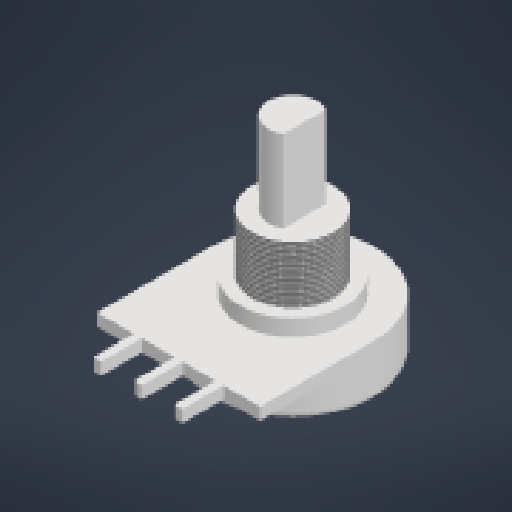
# Autodesk Inventor part: PotMeter
Saved by Autodesk Inventor 2026.1 (Build 301233000, 233)
## iProperties
Created: 2025-11-11
Part Number: PotMeter
Material: Generic
Document SubType Name: Modeling
Designer: Mikke
Density: 1 g/cm^3
Appearance: Default
Author: Mikke
Autodesk Inventor part; units mm, degrees
ref_plane "YZ Plane" through (0, 0, 0) normal (1, 0, 0) x (0, 1, 0)
ref_plane "XZ Plane" through (0, 0, 0) normal (0, 1, 0) x (-1, 0, 0)
ref_plane "XY Plane" through (0, 0, 0) normal (0, 0, 1) x (1, 0, 0)
sketch "Sketch1" plane through (0, 0, 0) normal (0, 1, 0) x (-1, 0, 0)
  circle A0 centre (0, 0) radius 10
  line L0 (10, 0) -> (-10, 0)
  line L1 (-10, 0) -> (-10, 14)
  line L2 (-10, 14) -> (10, 14)
  line L3 (10, 14) -> (10, 0)
  line L4 (-5.5, 14) -> (-4.5, 14)
  line L5 (-0.5, 14) -> (0.5, 14)
  line L6 (4.5, 14) -> (5.5, 14)
  line L7 (5.5, 14) -> (4.5, 14)
  line L8 (4.5, 14) -> (4.5, 19)
  line L9 (4.5, 19) -> (5.5, 19)
  line L10 (5.5, 19) -> (5.5, 14)
  line L11 (0.5, 14) -> (-0.5, 14)
  line L12 (-0.5, 14) -> (-0.5, 19)
  line L13 (-0.5, 19) -> (0.5, 19)
  line L14 (0.5, 19) -> (0.5, 14)
  line L15 (-4.5, 14) -> (-5.5, 14)
  line L16 (-5.5, 14) -> (-5.5, 19)
  line L17 (-5.5, 19) -> (-4.5, 19)
  line L18 (-4.5, 19) -> (-4.5, 14)
  point P0 (0, 14)
  point P1 (5, 14)
  point P2 (-5, 14)
  dimension "d0" = 20
  dimension "d1" = 20
  dimension "d2" = 14
  dimension "d5" = 1
  dimension "d6" = 1
  dimension "d7" = 1
  dimension "d8" = 5
  dimension "d9" = 5
  dimension "d10" = 5
  constraints: 38 end point, 8 parallel, 7 coincident, 5 point on line, 4 horizontal, 4 midpoint, 4 perpendicular, 3 other
  measures "d1" distance of L1.end L2.end
  measures "d2" distance of L0.end L1.end
  measures "d5" distance of L4.start L4.end
  measures "d6" distance of L5.start L5.end
  measures "d7" distance of L6.start L6.end
  measures "d8" distance of L7.end L8.end
  measures "d9" distance of L11.end L12.end
  measures "d10" distance of L15.end L16.end
extrude "Extrusion1" add sketch "Sketch1" along normal blind 1.5
sketch "Sketch2" plane through (0, 0, 0) normal (0, -1, 0) x (1, 0, 0)
  circle A0 centre (0, 0) radius 10
  constraints: 1 centre point, 1 coincident
extrude "Extrusion2" add sketch "Sketch2" along normal blind 5
sketch "Sketch3" plane through (0, 1.5, 0) normal (0, 1, 0) x (1, 0, 0)
  circle A0 centre (0, 0) radius 6.5
  dimension "d13" = 13
  constraints: 1 centre point, 1 coincident
  measures "d13" diameter of A0
extrude "Extrusion3" add sketch "Sketch3" along normal blind 2
sketch "Sketch4" plane through (0, 3.5, 0) normal (0, 1, 0) x (1, 0, 0)
  circle A0 centre (0, 0) radius 5
  dimension "d16" = 10
  constraints: 1 centre point, 1 coincident
  measures "d16" diameter of A0
extrude "Extrusion4" add sketch "Sketch4" along normal blind 7
thread "Thread1" size "M3x0.5" class "6g" standard "ANSI Metric M Profile" full length
sketch "Sketch5" plane through (0, 10.5, 0) normal (0, 1, 0) x (1, 0, 0)
  circle A0 centre (0, 0) radius 3
  line L0 (0, 0) -> (1.5, 0)
  line L1 (1.5, -2.5981) -> (1.5, 2.5981)
  point P0 (0.0162, 1.5)
  point P1 (-2.4, 1.8)
  dimension "d21" = 6
  dimension "d27" = 1.5
  constraints: 4 end point, 2 point on circle, 1 centre point, 1 coincident, 1 horizontal, 1 midpoint, 1 vertical
  measures "d21" diameter of A0
  measures "d27" distance of L0.start L0.end
extrude "Extrusion5" add sketch "Sketch5" along normal blind 10 contours L1 A0 picked at (-1.4848, 0)
fillet "Fillet1" radius 1 1 edges at (-10, -5, 0)
fillet "Fillet2" radius 0.2 6 edges at (5.5, 0.75, 19) (4.5, 0.75, 19) (0.5, 0.75, 19) (-0.5, 0.75, 19) (-4.5, 0.75, 19) (-5.5, 0.75, 19)
body "Solid1"
